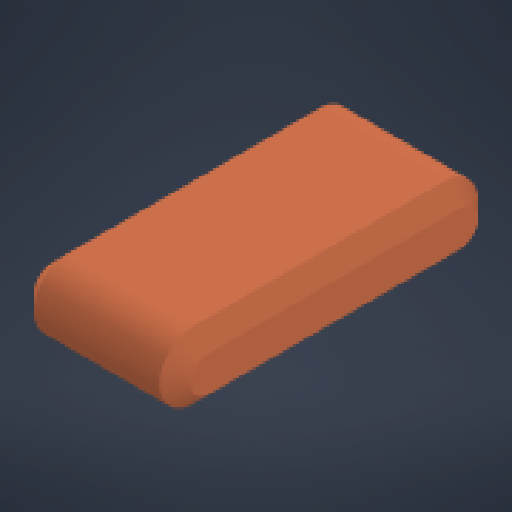
# Autodesk Inventor part: battery
Saved by Autodesk Inventor 2025.2 (Build 292293000, 293)
## iProperties
Created: 2025-07-12
Part Number: battery
Material: Generic
Document SubType Name: Modeling
Designer: micyg
Density: 1 g/cm^3
Appearance: Default
Author: micyg
Autodesk Inventor part; units mm, degrees
ref_plane "YZ Plane" through (0, 0, 0) normal (1, 0, 0) x (0, 1, 0)
ref_plane "XZ Plane" through (0, 0, 0) normal (0, 1, 0) x (-1, 0, 0)
ref_plane "XY Plane" through (0, 0, 0) normal (0, 0, 1) x (1, 0, 0)
sketch "Sketch1" plane through (0, 0, 0) normal (0, 1, 0) x (-1, 0, 0)
  line L0 (0, 0) -> (20, 0)
  line L1 (20, 0) -> (20, -40.5)
  line L2 (20, -40.5) -> (0, -40.5)
  line L3 (0, -40.5) -> (0, 0)
  dimension "d0" = 20
  dimension "d1" = 40.5
  constraints: 8 end point, 2 parallel, 1 horizontal, 1 perpendicular
  measures "d0" distance of L1.end L2.end
  measures "d1" distance of L0.end L1.end
extrude "Extrusion1" add sketch "Sketch1" along normal blind 8.5
fillet "Fillet1" radius 4.25 4 edges at (-10, 8.5, 0) (-10, 0, 0) (-10, 8.5, -40.5) (-10, 0, -40.5)
chamfer "Chamfer1" distance 2 angle 45 8 edges at (0, 8.5, -20.25) (0, 7.2554, -39.2554) (0, 0, -20.25) (0, 7.2554, -1.2446) (-20, 8.5, -20.25) (-20, 7.2554, -1.2446) (-20, 0, -20.25) (-20, 7.2554, -39.2554)
equation "\"d4\" = 0.5 * d2"
equation "\"d2\" = 8.5"
body "Solid1"
